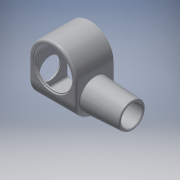
# Autodesk Inventor part: casting2
Saved by Autodesk Inventor 2019 (Build 230136000, 136)
## iProperties
Shininess: 20.0
Length Units: 11272
Angle Units: 11279
Time Units: 11290
Mass Units: 11286
Length Display Precision: 3
Angle Display Precision: 2
Compacted: True
Created: 2001-07-10
Part Number: casting2
Document SubType Name: Modeling
Designer: Autodesk, Inc.
Mass: 2.85472 g
Surface Area: 23.8543 cm^2
Volume: 1.0534 cm^3
Density: 2.71 g/cm^3
Material: Aluminum-6061
Appearance: Aluminum - Flat
Density: 0.0
Volumn: 0.0
Area: 0.0
PropertySet Name: Model Information
Control State: 0
Master: False
Checked Out: False
Author: Autodesk, Inc.
Autodesk Inventor part; units mm, degrees
ref_plane "YZ Plane" through (0, 0, 0) normal (1, 0, 0) x (0, 1, 0)
ref_plane "XZ Plane" through (0, 0, 0) normal (0, 1, 0) x (-1, 0, 0)
ref_plane "XY Plane" through (0, 0, 0) normal (0, 0, 1) x (1, 0, 0)
sketch "Sketch1" plane through (0, 0, 0) normal (0, 0, 1) x (1, 0, 0)
  line L0 (0, 12.7) -> (0, 0)
  line L1 (0, 0) -> (15.875, 0)
  line L2 (15.875, 0) -> (15.875, 12.7)
  arc A0 (15.875, 12.7) -> (0, 12.7) centre (7.9375, 12.7) ccw
  constraints: 6 end point, 2 point on circle, 1 centre point, 1 parallel, 1 perpendicular, 1 tangent, 1 vertical
extrude "Extrusion1" add sketch "Sketch1" along normal blind 12.7
fillet "Fillet7" radius 6.35 1 edges at (7.9375, 0, 12.7)
shell "Shell1" thickness 0.7937 removed faces 1 at (5.2917, 8.4667, 0)
sketch "Sketch2" plane through (0, 0, 0) normal (0, 0, -1) x (-1, 0, 0)
  line L0 (0, 0) -> (-15.875, 0) projected
  line L1 (0, 12.7) -> (0, 0) projected
  line L2 (0, 0) -> (0, -4.7625)
  arc A0 (-4.7625, -4.7625) -> (0, -4.7625) centre (-2.3813, -4.7625) ccw
  line L3 (-4.7625, -4.7625) -> (-4.7625, 0)
  constraints: 4 end point, 2 point on circle, 2 tangent, 1 centre point, 1 collinear, 1 perpendicular, 1 point on line
extrude "Extrusion2" add sketch "Sketch2" against normal blind 2.286
fillet "Fillet1" radius 0.762 1 edges at (2.3813, 0, 2.286)
fillet "Fillet2" radius 0.762 2 edges at (4.7625, 0, 2.667) (4.7625, 0, 1.143)
fillet "Fillet3" radius 0.762 10 edges at (0, 0, 4.699) (0, -0.2232, 2.5092) (0, -2.7623, 2.286) (2.3812, -7.1438, 2.286) (4.7625, -2.7622, 2.286) (4.9857, -0.2232, 2.5092) (15.875, 0, 3.175) (15.875, 9.525, 12.7) (7.9375, 20.6375, 12.7) (0, 9.525, 12.7)
sketch "Sketch3" plane through (0, 0, 2.286) normal (0, 0, 1) x (1, 0, 0)
  circle A0 centre (2.3813, -4.7625) radius 1.143
  line L0 (0, -0.762) -> (0, -4.7625) projected
  dimension "d10" = 2.3813
  dimension "d11" = 2.286
  constraints: 1 centre point
  measures "d10" distance from line of A0.centre L0
  measures "d11" diameter of A0
extrude "Extrusion3" cut sketch "Sketch3" against normal through all
fillet "Fillet8" radius 0.762 7 edges at (0.7937, 0.7937, 3.175) (0.7937, 2.4211, 10.2789) (0.7937, 9.525, 11.9062) (7.9375, 19.8438, 11.9062) (15.0813, 9.525, 11.9062) (15.0813, 2.4211, 10.2789) (15.0813, 0.7937, 3.175)
sketch "Sketch5" plane through (0, 0, 0) normal (0, 0, -1) x (-1, 0, 0)
  line L0 (-15.0812, 1.5558) -> (-15.0812, 12.7) projected
  arc A0 (-0.7937, 12.7) -> (-15.0812, 12.7) centre (-7.9375, 12.7) ccw projected
  line L1 (-0.7937, 12.7) -> (-0.7937, 1.5558) projected
  line L2 (-1.5558, 0.7937) -> (-14.3193, 0.7937) projected
  arc A1 (-1.5558, 0.7937) -> (-0.7937, 1.5558) centre (-1.5558, 1.5558) ccw projected
  arc A2 (-15.0812, 1.5558) -> (-14.3193, 0.7937) centre (-14.3193, 1.5558) ccw projected
  line L3 (-15.4781, 12.7) -> (-15.4781, 1.5557)
  arc A3 (-15.4781, 1.5557) -> (-14.3193, 0.3969) centre (-14.3193, 1.5558) ccw
  line L4 (-14.3193, 0.3969) -> (-1.5557, 0.3969)
  arc A4 (-1.5557, 0.3969) -> (-0.3969, 1.5558) centre (-1.5558, 1.5558) ccw
  line L5 (-0.3969, 1.5558) -> (-0.3969, 12.7)
  arc A5 (-0.3969, 12.7) -> (-15.4781, 12.7) centre (-7.9375, 12.7) ccw
  dimension "d53" = 0.3969
  constraints: 6 end point, 6 point on circle, 3 centre point, 5 other
  measures "d53" distance between parallel lines of L3 L0
extrude "Extrusion5" cut sketch "Sketch5" against normal blind 0.7937 contours L0 A0 L1 A1 L2 A2 | A5 L5 A4 L4 A3 L3
sketch "Sketch6" plane through (0, 0, 12.7) normal (0, 0, 1) x (1, 0, 0)
  circle A0 centre (7.9375, 12.7) radius 6.35
  line L0 (0, 12.7) -> (0, 0.762) projected
  dimension "d21" = 7.9375
  dimension "d28" = 12.7
  constraints: 1 centre point
  measures "d21" distance from line of A0.centre L0
  measures "d28" diameter of A0
extrude "Extrusion6" cut sketch "Sketch6" against normal through all
sketch "Sketch7" plane through (0, 0, 12.7) normal (0, 0, 1) x (1, 0, 0)
  circle A0 centre (7.9375, 12.7) radius 6.35 projected
  circle A1 centre (7.9375, 12.7) radius 6.7469
  dimension "d25" = 0.3969
  constraints: 1 centre point, 1 coincident
  measures "d25" radial gap between concentric circles of A0 A1
extrude "Extrusion7" cut sketch "Sketch7" against normal blind 0.3969
sketch "Sketch8" plane through (15.875, 0.762, 0) normal (1, 0, 0) x (0, 0, -1)
  circle A0 centre (-6.35, 5.588) radius 5.08
  line L0 (0, 0) -> (-6.35, 0) projected
  line L1 (0, 0) -> (0, 11.938) projected
  line L2 (0, 11.938) -> (-11.938, 11.938) projected
  line L3 (-11.938, 5.588) -> (-11.938, 11.938) projected
  arc A1 (-11.938, 5.588) -> (-6.35, 0) centre (-6.35, 5.588) ccw projected
  constraints: 1 centre point
extrude "Extrusion8" add sketch "Sketch8" along normal blind 12.7 draft -3 contours A0
fillet "Fillet5" radius 0.381 1 edges at (15.875, 6.35, 11.43)
fillet "Fillet6" radius 0.381 1 edges at (28.575, 6.35, 10.7644)
sketch "Sketch9" plane through (28.575, 6.35, 6.35) normal (1, 0, 0) x (0, 0, -1)
  circle A0 centre (0, 0) radius 4.0529 projected
  circle A1 centre (0, 0) radius 3.5719
  dimension "d36" = 7.1437
  constraints: 1 centre point, 1 coincident
  measures "d36" diameter of A1
extrude "Extrusion9" cut sketch "Sketch9" against normal through all contours A1
chamfer "Chamfer2" distance 0.254 angle 45 1 edges at (28.575, 6.35, 9.9219)
sketch "Sketch10" plane through (0, -4.7625, 0) normal (-1, 0, 0) x (0, 0, 1)
  circle A0 centre (6.35, 11.1125) radius 3.5719 projected
  circle A1 centre (6.35, 11.1125) radius 3.9688
  dimension "d43" = 7.9375
  constraints: 1 centre point, 1 coincident
  measures "d43" diameter of A1
extrude "Extrusion10" cut sketch "Sketch10" against normal blind 0.3969
chamfer "Chamfer5" distance 0.127 angle 45 6 edges at (7.9375, 20.2406, 0) (0.3969, 7.1279, 0) (0.7363, 0.7363, 0) (7.9375, 0.3969, 0) (15.1387, 0.7363, 0) (15.4781, 7.1279, 0)
chamfer "Chamfer6" distance 0.127 angle 45 1 edges at (1.1906, 12.7, 12.3031)
body "Solid1"
